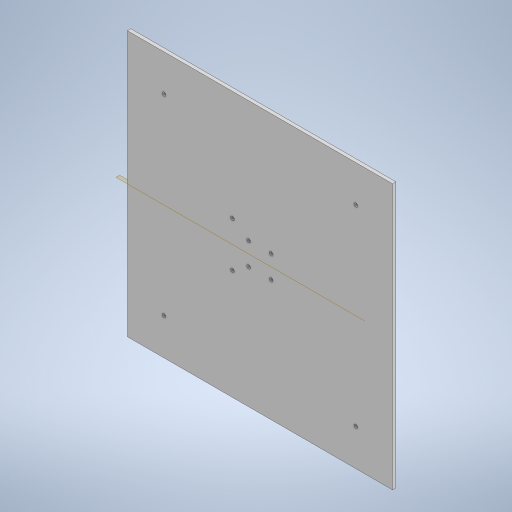
# Autodesk Inventor part: print bed base
Saved by Autodesk Inventor 2023.1 (Build 271208000, 208)
## iProperties
Created: 2022-10-30
Part Number: print bed base
Material: Generic
Document SubType Name: Modeling
Designer: nicol
Density: 1 g/cm^3
Appearance: Default
Author: nicol
Autodesk Inventor part; units mm, degrees
ref_plane "YZ Plane" through (0, 0, 0) normal (1, 0, 0) x (0, 1, 0)
ref_plane "XZ Plane" through (0, 0, 0) normal (0, 1, 0) x (-1, 0, 0)
ref_plane "XY Plane" through (0, 0, 0) normal (0, 0, 1) x (1, 0, 0)
sketch "Sketch1" plane through (0, 0, 0) normal (0, 0, 1) x (1, 0, 0)
  line L0 (0, 0) -> (234.95, 0)
  line L1 (234.95, 0) -> (234.95, 234.95)
  line L2 (234.95, 234.95) -> (0, 234.95)
  line L3 (0, 234.95) -> (0, 0)
  dimension "d0" = 234.95
  dimension "d1" = 234.95
  constraints: 8 end point, 2 parallel, 1 horizontal, 1 perpendicular
  measures "d0" distance of L2.end L1.end
  measures "d1" distance of L1.end L0.end
extrude "Extrusion1" add sketch "Sketch1" along normal blind 3
ref_plane "Work Plane1" through (0, 117.475, 0) normal (0, 1, 0) x (1, 0, 0)
sketch "Sketch2" plane through (0, 0, 3) normal (0, 0, 1) x (1, 0, 0)
  line L0 (0, 234.95) -> (0, 0) projected
  line L1 (234.95, 0) -> (234.95, 234.95) projected
  line L2 (0, 0) -> (234.95, 0) projected
  line L3 (234.95, 234.95) -> (0, 234.95) projected
  line L4 (54.825, 126.475) -> (78.825, 126.475) construction
  line L5 (156.125, 126.475) -> (180.125, 126.475) construction
  line L6 (107.475, 127.475) -> (127.475, 127.475) construction
  line L7 (127.475, 127.475) -> (127.475, 107.475) construction
  line L8 (127.475, 107.475) -> (107.475, 107.475) construction
  line L9 (107.475, 107.475) -> (107.475, 127.475) construction
  line L10 (93.15, 137.475) -> (93.15, 97.475) construction
  point P0 (32.475, 202.475)
  point P1 (202.475, 202.475)
  point P2 (202.475, 32.475)
  point P3 (32.475, 32.475)
  point P4 (54.825, 108.475)
  point P5 (78.825, 108.475)
  point P6 (156.125, 108.475)
  point P7 (180.125, 108.475)
  point P8 (66.825, 126.475)
  point P9 (168.125, 126.475)
  point P10 (117.475, 127.475)
  point P11 (117.475, 234.95)
  point P12 (127.475, 117.475)
  point P13 (234.95, 117.475)
  point P14 (93.15, 117.475)
  point P15 (0, 117.475)
  dimension "d4" = 170
  dimension "d5" = 170
  dimension "d6" = 32.475
  dimension "d7" = 32.475
  dimension "d8" = 32.475
  dimension "d9" = 32.475
  dimension "d17" = 24
  dimension "d18" = 18
  dimension "d19" = 18
  dimension "d20" = 24
  dimension "d21" = 101.3
  dimension "d22" = 54.825
  dimension "d23" = 54.825
  dimension "d24" = 108.475
  dimension "d25" = 108.475
  dimension "d33" = 20
  dimension "d34" = 40
  dimension "d35" = 14.325
  dimension "d36" = 14.325
  constraints: 14 end point, 8 horizontal alignment, 8 midpoint, 7 vertical alignment, 4 coincident, 3 horizontal, 2 parallel, 2 perpendicular, 1 collinear, 1 vertical
  measures "d4" distance of point (32.475, 202.475) point (202.475, 202.475)
  measures "d5" distance of point (202.475, 32.475) point (202.475, 202.475)
  measures "d6" distance from line of L0 point (32.475, 202.475)
  measures "d7" distance from line of L1 point (202.475, 202.475)
  measures "d8" distance from line of L2 point (202.475, 32.475)
  measures "d9" distance from line of L3 point (202.475, 202.475)
  measures "d17" distance of L5.end L5.start
  measures "d18" distance of point (180.125, 108.475) L5.end
  measures "d19" distance of point (78.825, 108.475) L4.end
  measures "d20" distance of L4.start L4.end
  measures "d21" distance of point (66.825, 126.475) point (168.125, 126.475)
  measures "d22" distance from line of L1 point (180.125, 108.475)
  measures "d23" distance from line of L0 point (54.825, 108.475)
  measures "d24" distance from line of L3 L5.end
  measures "d25" distance from line of L2 point (180.125, 108.475)
  measures "d33" distance of L6.start L6.end
  measures "d34" distance of L10.start L10.end
  measures "d35" distance from line of point (107.475, 127.475) L10
  measures "d36" distance from line of L4.end L10
hole "Hole1" at (32.475, 202.475, 3) at (202.475, 202.475, 3) at (202.475, 32.475, 3) at (32.475, 32.475, 3) at (107.475, 127.475, 3) at (127.475, 127.475, 3) at (127.475, 107.475, 3) at (107.475, 107.475, 3) at (93.15, 137.475, 3) at (93.15, 97.475, 3) direction (0, 0, -1) diameter 3.2 end through all
equation "\"d5\" = d4"
equation "\"d6\" = d7"
equation "\"d8\" = d9"
equation "\"d19\" = d18"
equation "\"d20\" = d17"
equation "\"d22\" = d23"
equation "\"d24\" = d25"
equation "\"d35\" = d36"
body "Solid1"
